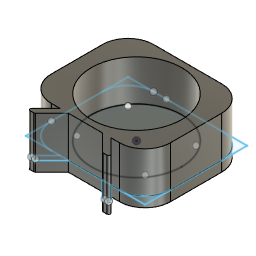
小米小电视音箱支架 (Autodesk Fusion 360 design; units mm, degrees)
Autodesk Fusion 360 part; units mm, degrees
sketch "草图1" plane through (0, 0, 0) normal (0, 0, 1) x (1, 0, 0)
  line L0 (-35, 30) -> (35, 30)
  line L1 (35, 30) -> (35, -30)
  line L2 (35, -30) -> (-35, -30)
  line L3 (-35, -30) -> (-35, 30)
  arc A0 (-20, 30) -> (-35, 15) centre (-20, 15) ccw
  arc A1 (-35, -15) -> (-20, -30) centre (-20, -15) ccw
  arc A2 (20, -30) -> (35, -15) centre (20, -15) ccw
  arc A3 (35, 15) -> (20, 30) centre (20, 15) ccw
  line L4 (-15, -30) -> (-23.2929, -38.2929)
  line L5 (-22.5858, -40) -> (-20.4142, -40)
  line L6 (-19.7071, -39.7071) -> (-10, -30)
  line L7 (10, -30) -> (19.7071, -39.7071)
  line L8 (20.4142, -40) -> (22.5858, -40)
  line L9 (23.2929, -38.2929) -> (15, -30)
  arc A4 (-23.2929, -38.2929) -> (-22.5858, -40) centre (-22.5858, -39) ccw
  arc A5 (-20.4142, -40) -> (-19.7071, -39.7071) centre (-20.4142, -39) ccw
  arc A6 (19.7071, -39.7071) -> (20.4142, -40) centre (20.4142, -39) ccw
  arc A7 (22.5858, -40) -> (23.2929, -38.2929) centre (22.5858, -39) ccw
  circle A8 centre (0, 0) radius 26.5
  line L10 (-12.4856, 30) -> (-10, 30)
  dimension "d2" = 60
  dimension "d3" = 70
  dimension "d4" = 1
  dimension "d5" = 1
  dimension "d6" = 1
  dimension "d7" = 1
  dimension "d8" = 53
  constraint horizontal L0
  constraint vertical L1
  constraint horizontal L2
  constraint vertical L3
  constraint coincident L3 A0.end
  constraint coincident L2 A1.end
  constraint coincident L1 A2.end
  constraint coincident L2 A2.start
  constraint coincident L0 A3.end
  constraint coincident L1 A3.start
  constraint coincident L2 L4.start
  constraint parallel L2 L5
  constraint coincident L2 L6.end
  constraint parallel L4 L6
  constraint coincident L2 L7.start
  constraint perpendicular L6 L7
  constraint parallel L2 L8
  constraint coincident L2 L9.end
  constraint parallel L7 L9
  constraint tangent L4 A4
  constraint tangent L5 A4
  constraint tangent L5 A5
  constraint tangent L6 A5
  constraint tangent L7 A6
  constraint tangent L8 A6
  constraint tangent L8 A7
  constraint tangent L9 A7
  constraint coincident A8.centre origin
  constraint coincident L0 L10.start
  constraint coincident L0 L10.end
  measures "d2" distance of L0 L2
  measures "d3" distance of L0 L5
  measures "d4" radius of A4
  measures "d5" radius of A5
  measures "d6" radius of A6
  measures "d7" radius of A7
  measures "d8" diameter of A8
extrude "拉伸1" add sketch "草图1" against normal blind 6 contours L0 L1 L2 L3 A0 A1 A2 A3 L10 | L2 L4 L5 L6 A4 A5 | L2 L7 L8 L9 A6 A7 | A8 makes body 1
extrude "拉伸2" add sketch "草图1" along normal blind 24 separate body contours L0 L1 L2 L3 A0 A1 A2 A3 L10 | L2 L4 L5 L6 A4 A5 | L2 L7 L8 L9 A6 A7 makes body 2
